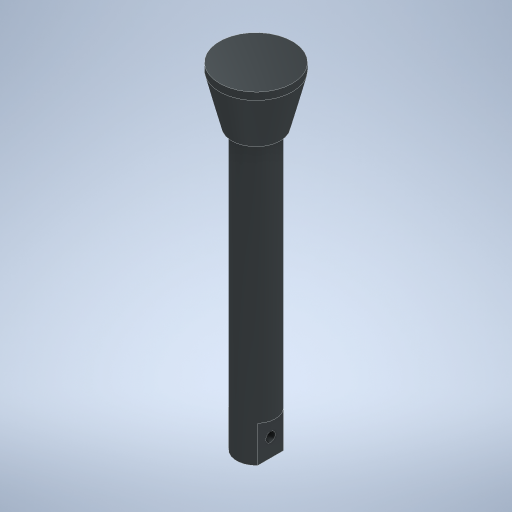
# Autodesk Inventor part: piston
Saved by Autodesk Inventor 2024.2 (Build 282272000, 272)
## iProperties
Created: 2024-05-29
Part Number: piston
Material: Iron, Ductile
Document SubType Name: Modeling
Designer: user
Density: 7.15 g/cm^3
Appearance: Iron Gray
Author: user
Autodesk Inventor part; units mm, degrees
ref_plane "YZ Plane" through (0, 0, 0) normal (1, 0, 0) x (0, 1, 0)
ref_plane "XZ Plane" through (0, 0, 0) normal (0, 1, 0) x (-1, 0, 0)
ref_plane "XY Plane" through (0, 0, 0) normal (0, 0, 1) x (1, 0, 0)
sketch "Sketch1" plane through (0, 0, 0) normal (0, 0, 1) x (1, 0, 0)
  line L0 (0, 0) -> (0, 138)
  line L1 (0, 138) -> (15, 138)
  line L2 (15, 138) -> (15, 135)
  line L3 (0, 0) -> (8, 0)
  line L4 (8, 0) -> (8, 115)
  line L5 (8, 115) -> (10, 115)
  line L6 (10, 115) -> (15, 135)
  line L7 (0, -27.6) -> (0, 165.6) projected
  dimension "d0" = 138
  dimension "d1" = 15
  dimension "d2" = 3
  dimension "d3" = 8
  dimension "d4" = 115
  dimension "d5" = 2
  constraints: 14 end point, 4 perpendicular, 1 horizontal, 1 vertical
  measures "d0" distance of L0.start L0.end
  measures "d1" distance of L0.end L1.end
  measures "d2" distance of L1.end L2.end
  measures "d3" distance of L0.start L3.end
  measures "d4" distance of L3.end L4.end
  measures "d5" distance of L4.end L5.end
revolve "Revolution1" add sketch "Sketch1" angle 360 about axis through (0, -10, 0) along (0, 1, 0)
sketch "Sketch2" plane through (0, 0, 0) normal (0, 0, 1) x (1, 0, 0)
  line L0 (8, 0) -> (-8, 0) projected
  line L1 (8, 15) -> (-8, 15)
  line L2 (-8, 15) -> (-6, 15)
  line L3 (-6, 15) -> (-6, 0)
  line L4 (-6, 0) -> (-8, 0)
  line L5 (-8, 0) -> (-8, 15)
  point P0 (0, 0)
  dimension "d7" = 15
  constraints: 10 end point, 3 parallel, 1 horizontal, 1 perpendicular, 1 point on line
  measures "d7" distance between parallel lines of L0 L1
extrude "Extrusion1" cut sketch "Sketch2" along normal through all both and the other way through all
mirror "Mirror1" about plane through (0, 0, 0) normal (1, 0, 0) of "Extrusion1"
sketch "Sketch3" plane through (6, 0, -5.2915) normal (1, 0, 0) x (0, 0, -1)
  line L0 (0, 15) -> (0, 0) projected
  line L1 (0, 15) -> (-10.583, 15) projected
  line L2 (-10.583, 0) -> (-10.583, 15) projected
  line L3 (0, 0) -> (-10.583, 0) projected
  circle A0 centre (-5.2915, 7.5) radius 2
  point P0 (-5.2915, 0)
  dimension "d10" = 4
  constraints: 1 centre point, 1 coincident
  measures "d10" diameter of A0
extrude "Extrusion2" cut sketch "Sketch3" against normal through all contours A0
body "Solid1"
